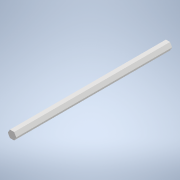
# Autodesk Inventor part: eje1_n
Saved by Autodesk Inventor 2022 (Build 260153000, 153)
## iProperties
Created: 2022-03-10
Part Number: eje1_n
Material: Generic
Document SubType Name: Modeling
Designer: katha
Density: 1 g/cm^3
Appearance: Default
Author: katha
Autodesk Inventor part; units mm, degrees
ref_plane "YZ Plane" through (0, 0, 0) normal (1, 0, 0) x (0, 1, 0)
ref_plane "XZ Plane" through (0, 0, 0) normal (0, 1, 0) x (-1, 0, 0)
ref_plane "XY Plane" through (0, 0, 0) normal (0, 0, 1) x (1, 0, 0)
sketch "Sketch1" plane through (0, 0, 0) normal (0, 0, 1) x (1, 0, 0)
  line L0 (0, 0) -> (3.1, 0) construction
  circle A0 centre (0, 0) radius 2.0286 construction
  line L1 (0, 0) -> (1.55, 2.6847) construction
  line L2 (0, 0) -> (-1.55, 2.6847) construction
  line L3 (0, 0) -> (-3.1, 0) construction
  line L4 (0, 0) -> (-1.55, -2.6847) construction
  line L5 (0, 0) -> (1.55, -2.6847) construction
  line L6 (-1.55, 2.6847) -> (1.55, 2.6847)
  line L7 (1.55, 2.6847) -> (3.1, 0)
  line L8 (3.1, 0) -> (1.55, -2.6847)
  line L9 (1.55, -2.6847) -> (-1.55, -2.6847)
  line L10 (-1.55, -2.6847) -> (-3.1, 0)
  line L11 (-3.1, 0) -> (-1.55, 2.6847)
  dimension "d0" = 3.1
  dimension "d3" = 360
  constraints: 24 end point, 3 parallel, 2 horizontal, 1 centre point, 1 coincident, 19 other
  measures "d0" distance of L0.start L0.end
extrude "Extrusion1" add sketch "Sketch1" along normal blind 115
sketch "Sketch2" plane through (-1.55, -2.6847, 0) normal (0, -1, 0) x (1, 0, 0)
  circle A0 centre (1.55, 5) radius 0.65
  line L0 (3.1, 0) -> (3.1, 115) projected
  line L1 (0, 0) -> (0, 115) projected
  line L2 (0, 0) -> (3.1, 0) projected
  circle A1 centre (1.55, 60) radius 0.65
  circle A2 centre (1.55, 57) radius 0.65
  point P0 (1.55, 0)
  point P1 (1.55, 0)
  dimension "d7" = 1.3
  dimension "d8" = 5
  dimension "d9" = 60
  dimension "d10" = 3
  constraints: 3 centre point, 3 vertical alignment, 2 equal radius, 1 midpoint
  measures "d7" diameter of A0
  measures "d8" distance of point (1.55, 0) A0.centre
  measures "d9" distance from line of L2 A1.centre
  measures "d10" distance of A2.centre A1.centre
extrude "Extrusion2" cut sketch "Sketch2" against normal blind 10
body "Solid1"
